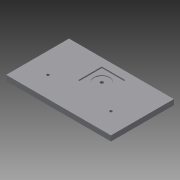
# Autodesk Inventor part: tractor
Saved by Autodesk Inventor 2013 (Build 170138000, 138)
## iProperties
Created: 2012-11-28
Part Number: tractor
Material: Generic
Document SubType Name: Modeling
Designer: Istvan
Density: 1 g/cm^3
Author: Istvan
Autodesk Inventor part; units mm, degrees
ref_plane "YZ Plane" through (0, 0, 0) normal (1, 0, 0) x (0, 1, 0)
ref_plane "XZ Plane" through (0, 0, 0) normal (0, 1, 0) x (-1, 0, 0)
ref_plane "XY Plane" through (0, 0, 0) normal (0, 0, 1) x (1, 0, 0)
sketch "Sketch1" plane through (0, 0, 0) normal (0, 1, 0) x (-1, 0, 0)
  line L0 (0, 0) -> (254, 0)
  line L1 (254, 0) -> (254, 152.4)
  line L2 (254, 152.4) -> (0, 152.4)
  line L3 (0, 152.4) -> (0, 0)
  dimension "d0" = 254
  dimension "d1" = 152.4
  constraints: 8 end point, 2 parallel, 1 horizontal, 1 perpendicular
  measures "d0" distance of L2.end L1.end
  measures "d1" distance of L1.end L0.end
extrude "Extrusion1" add sketch "Sketch1" against normal blind 12.7
sketch "Sketch2" plane through (0, 0, 0) normal (0, 1, 0) x (1, 0, 0)
  line L0 (0, 0) -> (-254, 0) projected
  line L1 (-254, 0) -> (-254, -152.4) projected
  line L2 (0, -152.4) -> (0, 0) projected
  line L3 (-155.575, -19.05) -> (-98.425, -19.05)
  line L4 (-98.425, -19.05) -> (-98.425, -76.2)
  line L5 (-98.425, -76.2) -> (-155.575, -76.2)
  line L6 (-155.575, -76.2) -> (-155.575, -19.05)
  dimension "d4" = 57.15
  dimension "d6" = 57.15
  dimension "d7" = 98.425
  dimension "d8" = 98.425
  dimension "d9" = 19.05
  constraints: 8 end point, 2 parallel, 1 horizontal, 1 perpendicular
  measures "d4" distance of L4.end L5.end
  measures "d6" distance of L3.end L4.end
  measures "d7" distance between parallel lines of L1 L6
  measures "d8" distance between parallel lines of L2 L4
  measures "d9" distance between parallel lines of L0 L3
extrude "Extrusion2" cut sketch "Sketch2" against normal blind 3.175
sketch "Sketch3" plane through (0, -3.175, 0) normal (0, 1, 0) x (1, 0, 0)
  line L0 (-98.425, -76.2) -> (-155.575, -76.2) projected
  line L1 (-98.425, -19.05) -> (-98.425, -76.2) projected
  circle A0 centre (-127, -47.625) radius 19.05
  point P0 (0, 0)
  dimension "d12" = 38.1
  dimension "d13" = 28.575
  dimension "d14" = 28.575
  constraints: 1 centre point
  measures "d12" diameter of A0
  measures "d13" distance from line of L0 A0.centre
  measures "d14" distance from line of L1 A0.centre
extrude "Extrusion3" cut sketch "Sketch3" against normal blind 1.524
sketch "Sketch4" plane through (-127, -4.699, 47.625) normal (0, 1, 0) x (1, 0, 0)
  circle A0 centre (0, 0) radius 19.05 projected
  circle A1 centre (0, 0) radius 3.81
  point P0 (127, 47.625)
  dimension "d17" = 7.62
  constraints: 1 centre point, 1 coincident
  measures "d17" diameter of A1
extrude "Extrusion4" cut sketch "Sketch4" against normal through all contours A1
sketch "Sketch5" plane through (0, -12.7, 0) normal (0, -1, 0) x (1, 0, 0)
  line L0 (0, 0) -> (0, 152.4) projected
  line L1 (0, 152.4) -> (-254, 152.4) projected
  line L2 (-254, 152.4) -> (-254, 0) projected
  point P0 (-50.8, 101.6)
  point P1 (-203.2, 101.6)
  dimension "d20" = 50.8
  dimension "d21" = 50.8
  dimension "d22" = 50.8
  constraints: 1 horizontal alignment
  measures "d20" distance from line of L1 point (-203.2, 101.6)
  measures "d21" distance from line of L2 point (-203.2, 101.6)
  measures "d22" distance from line of L0 point (-50.8, 101.6)
hole "Hole1" at (-50.8, -12.7, 101.6) at (-203.2, -12.7, 101.6) direction (0, 1, 0) diameter 6.35 end through all
equation "\"d7\" = d8"
equation "\"d22\" = d21"
body "Solid1"
